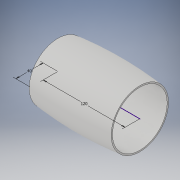
# Autodesk Inventor part: sugardrum1
Saved by Autodesk Inventor 2019 (Build 230136000, 136)
## iProperties
Created: 2020-02-19
Part Number: sugardrum1
Material: Generic
Document SubType Name: Modeling
Designer: ACHYUTH
Density: 1 g/cm^3
Appearance: Default
Author: ACHYUTH
Autodesk Inventor part; units mm, degrees
ref_plane "YZ Plane" through (0, 0, 0) normal (1, 0, 0) x (0, 1, 0)
ref_plane "XZ Plane" through (0, 0, 0) normal (0, 1, 0) x (-1, 0, 0)
ref_plane "XY Plane" through (0, 0, 0) normal (0, 0, 1) x (1, 0, 0)
sketch "Sketch1" plane through (0, 0, 0) normal (0, 1, 0) x (-1, 0, 0)
  line L0 (0, 0) -> (0, 40)
  line L1 (0, 40) -> (120, 40)
  line L2 (120, 40) -> (120, 42)
  line L3 (0, 40) -> (0, 42)
  arc A0 (120, 40) -> (0, 40) centre (60, -501.1279) ccw
  arc A1 (120, 42) -> (0, 42) centre (60, -499.1279) ccw
  line L4 (144, 0) -> (-24, 0) projected
  dimension "d0" = 40
  dimension "d1" = 120
  dimension "d2" = 2
  dimension "d3" = 2
  constraints: 8 end point, 4 point on circle, 3 vertical, 2 centre point, 1 equal radius, 1 horizontal
  measures "d0" distance of L0.start L0.end
  measures "d1" distance of L0.end L1.end
  measures "d2" distance of L1.end L2.end
  measures "d3" distance of L0.end L3.end
sketch "Sketch2" plane through (0, 0, 0) normal (0, 1, 0) x (-1, 0, 0)
  line L0 (0, 0) -> (120, 0)
  line L1 (120, 0) -> (120, 40)
  dimension "d4" = 120
  dimension "d5" = 40
  constraints: 4 end point, 1 horizontal, 1 perpendicular
  measures "d4" distance of L0.start L0.end
  measures "d5" distance of L0.end L1.end
revolve "Revolution1" add sketch "Sketch1" angle 360 about axis through (-10, 0, 0) along (1, 0, 0) contours L3 A1 L2 A0
body "Solid1"
